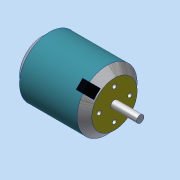
# Autodesk Inventor part: TurnigySK3_Mock
Saved by Autodesk Inventor 2015 SP1 (Build 190203100, 203)
## iProperties
Created: 2015-06-15
Part Number: TurnigySK3_Mock
Material: Aluminum 6061
Document SubType Name: Modeling
Designer: YOUR_NAME_HERE
Density: 2.7 g/cm^3
Appearance: Aluminum - Flat
Author: YOUR_NAME_HERE
Autodesk Inventor part; units mm, degrees
ref_plane "YZ Plane" through (0, 0, 0) normal (1, 0, 0) x (0, 1, 0)
ref_plane "XZ Plane" through (0, 0, 0) normal (0, 1, 0) x (-1, 0, 0)
sketch "Sketch1" plane through (0, 0, 0) normal (1, 0, 0) x (0, 1, 0)
  circle A0 centre (0, 0) radius 24.5
  dimension "d0" = 49
  constraints: 1 centre point, 1 coincident
  measures "d0" diameter of A0
extrude "Extrusion1" add sketch "Sketch1" along normal blind 59
sketch "Sketch2" plane through (59, 0, 0) normal (1, 0, 0) x (0, 0, -1)
  circle A0 centre (0, 0) radius 3
  dimension "d3" = 6
  constraints: 1 centre point, 1 coincident
  measures "d3" diameter of A0
extrude "Extrusion2" add sketch "Sketch2" along normal blind 21
sketch "Sketch3" plane through (59, 0, 0) normal (1, 0, 0) x (0, 0, -1)
  circle A0 centre (0, 0) radius 12.5 construction
  circle A1 centre (0, 12.5) radius 1.65
  circle A2 centre (12.5, 0) radius 1.65
  circle A3 centre (0, -12.5) radius 1.65
  circle A4 centre (-12.5, 0) radius 1.65
  line L0 (0, -34.3) -> (0, 34.3) projected
  line L1 (-34.3, 0) -> (34.3, 0) projected
  dimension "d6" = 25
  dimension "d7" = 3.3
  constraints: 5 centre point, 4 point on circle, 4 point on line, 3 equal radius, 1 coincident
  measures "d6" diameter of A0
  measures "d7" diameter of A1
extrude "Extrusion3" cut sketch "Sketch3" against normal through all
chamfer "Chamfer1" distance 6 angle 45 2 edges at (59, -24.5, 0) (0, -24.5, 0)
ref_plane "Work Plane2" through (0, 0, 0) normal (0, -0.7071, 0.7071) x (1, 0, 0)
sketch "Sketch5" plane through (0, 0, 0) normal (0, -0.7071, 0.7071) x (1, 0, 0)
  line L0 (53, -24.5) -> (53, 24.5) projected
  line L1 (59, 18.5) -> (59, -18.5) projected
  line L2 (53, 24.5) -> (59, 18.5) projected
  line L3 (53, -24.5) -> (59, -18.5) projected
  line L4 (54.0835, 23.4165) -> (54.0835, 33.5765)
  line L5 (54.0835, 33.5765) -> (58.4015, 33.5765)
  line L6 (58.4015, 33.5765) -> (58.4015, 19.0985)
  point P0 (0, 0)
  dimension "d19" = 10.16
  dimension "d21" = 4.318
  dimension "d22" = 1.0835
  constraints: 6 end point, 2 perpendicular, 2 point on line, 1 vertical
  measures "d19" distance from line of L4.start L5
  measures "d21" distance between parallel lines of L6 L4
  measures "d22" distance from line of L0.end L4
extrude "Extrusion5" add sketch "Sketch5" along normal mid plane 7.62 contours L4 L5 L6 L2
body "Solid1"
